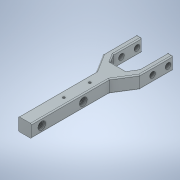
# Autodesk Inventor part: basisachse
Saved by Autodesk Inventor 2022 (Build 260153000, 153)
## iProperties
Created: 2022-02-25
Part Number: basisachse
Material: Generisch
Document SubType Name: Modeling
Designer: 123St
Density: 1 g/cm^3
Appearance: Zink
Author: 123St
Autodesk Inventor part; units mm, degrees
ref_plane "YZ Plane" through (0, 0, 0) normal (1, 0, 0) x (0, 1, 0)
ref_plane "XZ Plane" through (0, 0, 0) normal (0, 1, 0) x (-1, 0, 0)
ref_plane "XY Plane" through (0, 0, 0) normal (0, 0, 1) x (1, 0, 0)
sketch "Skizze1" plane through (0, 0, 0) normal (0, 1, 0) x (-1, 0, 0)
  line L0 (-12.5, 19.9585) -> (-35, -16.0415)
  line L1 (-35, -16.0415) -> (-35, -81.0415)
  line L2 (-35, -81.0415) -> (-25, -81.0415)
  line L3 (-25, -81.0415) -> (-25, -26.0415)
  line L4 (-25, -26.0415) -> (-15, -10.0415)
  line L5 (-15, -10.0415) -> (15, -10.0415)
  line L6 (15, -10.0415) -> (25, -26.0415)
  line L7 (25, -26.0415) -> (25, -81.0415)
  line L8 (25, -81.0415) -> (35, -81.0415)
  line L9 (35, -81.0415) -> (35, -16.0415)
  line L10 (35, -16.0415) -> (12.5, 19.9585)
  line L11 (0, -101.2415) -> (0, 40.1585) projected
  line L12 (12.5, 19.9585) -> (-12.5, 19.9585)
  point P0 (0, 0)
  dimension "d0" = 10
  dimension "d1" = 10
  dimension "d4" = 30
  dimension "d5" = 15
  dimension "d6" = 70
  dimension "d7" = 55
  dimension "d8" = 55
  dimension "d9" = 65
  dimension "d10" = 65
  dimension "d11" = 10
  dimension "d13" = 25
  dimension "d14" = 30
  dimension "d15" = 30
  dimension "d16" = 50
  constraints: 24 end point, 4 perpendicular, 3 parallel, 2 point on line
  measures "d0" distance of L7.end L8.end
  measures "d1" distance of L1.end L2.end
  measures "d4" distance of L4.end L5.end
  measures "d5" distance from line of L11 L5.end
  measures "d6" distance between parallel lines of L1 L9
  measures "d7" distance of L6.end L7.end
  measures "d8" distance of L2.end L3.end
  measures "d9" distance of L8.end L9.end
  measures "d10" distance of L0.end L1.end
  measures "d11" horizontal distance of L5.end L6.end
  measures "d13" distance of L10.end L0.start
  measures "d14" vertical distance of L0.start L4.end
  measures "d15" vertical distance of L10.end L5.end
  measures "d16" distance of L7.end L2.end
extrude "Extrusion1" add sketch "Skizze1" along normal blind 25
sketch "Skizze2" plane through (-12.5, 0, 19.9585) normal (0, 0, 1) x (1, 0, 0)
  line L0 (-22.5, 25) -> (0, 25) projected
  line L1 (0, 0) -> (25, 0) projected
  line L2 (0, 25) -> (25, 25)
  line L3 (25, 25) -> (25, 0)
  line L4 (25, 0) -> (0, 0)
  line L5 (0, 0) -> (0, 25)
  point P0 (12.5, 0)
  constraints: 8 end point, 2 parallel, 1 horizontal, 1 perpendicular
extrude "Extrusion2" add sketch "Skizze2" along normal blind 150
sketch "Skizze3" plane through (35, 0, -16.0415) normal (1, 0, 0) x (0, 0, -1)
  circle A0 centre (55, 12.5) radius 5.5
  circle A1 centre (25, 12.5) radius 5.5
  line L0 (-236.2, 0) -> (115.2, 0) projected
  line L1 (65, 0) -> (65, 25) projected
  point P0 (-16.0415, 0)
  dimension "d21" = 12.5
  dimension "d22" = 12.5
  dimension "d23" = 30
  dimension "d24" = 11
  dimension "d25" = 11
  dimension "d26" = 10
  constraints: 2 centre point
  measures "d21" distance from line of L0 A0.centre
  measures "d22" distance from line of L0 A1.centre
  measures "d23" distance of A0.centre A1.centre
  measures "d24" diameter of A0
  measures "d25" diameter of A1
  measures "d26" distance from line of L1 A0.centre
extrude "Extrusion3" cut sketch "Skizze3" against normal blind 300
fillet "Rundung1" radius 2 30 edges at (-20, 25, -18.0415) (0, 25, -10.0415) (-25, 25, -53.5415) (20, 25, -18.0415) (25, 25, -53.5415) (30, 25, -81.0415) (-30, 25, -81.0415) (-35, 25, -48.5415) (-23.75, 25, 1.9585) (23.75, 25, 1.9585) (12.5, 25, 94.9585) (-12.5, 25, 94.9585) (-25, 12.5, -81.0415) (-35, 12.5, -81.0415) (25, 12.5, -81.0415) (35, 12.5, -81.0415) (35, 25, -48.5415) (30, 0, -81.0415) (35, 0, -48.5415) (25, 0, -53.5415) (20, 0, -18.0415) (0, 0, -10.0415) (-20, 0, -18.0415) (-25, 0, -53.5415) (-30, 0, -81.0415) (-35, 0, -48.5415) (23.75, 0, 1.9585) (-23.75, 0, 1.9585) (-12.5, 0, 94.9585) (12.5, 0, 94.9585)
sketch "Skizze4" plane through (12.5, 2, 169.9585) normal (1, 0, 0) x (0, 0, -1)
  circle A0 centre (20, 10) radius 5
  circle A1 centre (100, 10) radius 5
  line L0 (0, 0) -> (0, 21) projected
  line L1 (0, -2) -> (150.5736, -2) projected
  point P0 (169.9585, -2)
  dimension "d31" = 10
  dimension "d32" = 10
  dimension "d33" = 20
  dimension "d34" = 80
  dimension "d35" = 12
  dimension "d36" = 12
  constraints: 2 centre point
  measures "d31" diameter of A0
  measures "d32" diameter of A1
  measures "d33" distance from line of L0 A0.centre
  measures "d34" distance of A0.centre A1.centre
  measures "d35" distance from line of L1 A0.centre
  measures "d36" distance from line of L1 A1.centre
extrude "Extrusion4" cut sketch "Skizze4" against normal blind 29
sketch "Skizze5" plane through (0, 0, 0) normal (0, -1, 0) x (1, 0, 0)
  circle A0 centre (0, 44.9585) radius 2.25
  circle A1 centre (0, 94.9585) radius 2.25
  line L0 (12.5, 19.9585) -> (12.5, 169.9585) projected
  line L1 (-10.5, 169.9585) -> (10.5, 169.9585) projected
  point P0 (0, 0)
  dimension "d39" = 4.5
  dimension "d40" = 4.5
  dimension "d41" = 50
  dimension "d42" = 12.5
  dimension "d43" = 12.5
  dimension "d44" = 75
  constraints: 2 centre point
  measures "d39" diameter of A1
  measures "d40" diameter of A0
  measures "d41" distance of A1.centre A0.centre
  measures "d42" distance from line of L0 A0.centre
  measures "d43" distance from line of L0 A1.centre
  measures "d44" distance from line of L1 A1.centre
extrude "Extrusion5" cut sketch "Skizze5" against normal blind 30
sketch "Skizze6" plane through (12.5, 2, 169.9585) normal (1, 0, 0) x (0, 0, -1)
  circle A0 centre (100, 10) radius 5 projected
  circle A1 centre (100, 10) radius 7.4925
  circle A2 centre (20, 10) radius 5 projected
  circle A3 centre (20, 10) radius 7.4925
  point P0 (169.9585, -2)
  dimension "d47" = 14.985
  dimension "d48" = 14.985
  constraints: 2 centre point, 2 coincident
  measures "d47" diameter of A1
  measures "d48" diameter of A3
extrude "Extrusion6" cut sketch "Skizze6" against normal blind 5
sketch "Skizze7" plane through (-12.5, 2, 19.9585) normal (-1, 0, 0) x (0, 0, 1)
  circle A0 centre (130, 10) radius 5 projected
  circle A1 centre (130, 10) radius 7.4925
  circle A2 centre (50, 10) radius 5 projected
  circle A3 centre (50, 10) radius 7.4925
  point P0 (-19.9585, -2)
  dimension "d51" = 14.985
  dimension "d52" = 14.985
  constraints: 2 centre point, 2 coincident
  measures "d51" diameter of A3
  measures "d52" diameter of A1
extrude "Extrusion7" cut sketch "Skizze7" against normal blind 5
